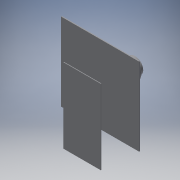
# Autodesk Inventor part: base1
Saved by Autodesk Inventor 2019 (Build 230136000, 136)
## iProperties
Created: 2019-05-27
Part Number: base1
Material: Generic
Document SubType Name: Modeling
Designer: felix
Density: 1 g/cm^3
Appearance: Default
Mass: 50923.6 g
Surface Area: 49527 cm^2
Volume: 50923.6 cm^3
Author: felix
Autodesk Inventor part; units mm, degrees
sketch "Sketch1" plane through (0, 0, 0) normal (0, 0, 1) x (1, 0, 0)
  circle A0 centre (0, 0) radius 130.5
  dimension "d0" = 261
  constraints: 1 centre point, 1 coincident
  measures "d0" diameter of A0
extrude "Extrusion1" add sketch "Sketch1" along normal blind 30 and the other way blind 95
sketch "Sketch2" plane through (0, 0, 30) normal (0, 0, 1) x (1, 0, 0)
  circle A0 centre (0, 0) radius 172.5
  dimension "d3" = 345
  constraints: 1 centre point, 1 coincident
  measures "d3" diameter of A0
extrude "Extrusion2" add sketch "Sketch2" along normal blind 125 and the other way blind 52.75
sketch "Sketch3" plane through (0, 0, 155) normal (0, 0, 1) x (1, 0, 0)
  line L0 (-920, 350) -> (330, 350)
  line L1 (330, 350) -> (330, -900)
  line L2 (330, -900) -> (-920, -900)
  line L3 (-920, -900) -> (-920, 350)
  point P0 (0, 0)
  dimension "d8" = 920
  dimension "d9" = 1250
  dimension "d10" = 900
  dimension "d11" = 1250
  constraints: 8 end point, 2 parallel, 1 horizontal, 1 perpendicular
  measures "d8" distance from line of point (0, 0) L3
  measures "d9" distance of L0.end L1.end
  measures "d10" vertical distance of point (0, 0) L2.end
  measures "d11" distance of L1.end L2.end
extrude "Extrusion3" add sketch "Sketch3" along normal blind 15
sketch "Sketch5" plane through (0, 0, 155) normal (0, 0, -1) x (-1, 0, 0)
  line L0 (-315, -885) -> (905, -885)
  line L1 (905, -885) -> (905, 335)
  line L2 (905, 335) -> (-315, 335)
  line L3 (-315, 335) -> (-315, -885)
  line L4 (590, -885) -> (590, -515)
  line L5 (590, -515) -> (905, -515)
  line L6 (590, -515) -> (590, -105)
  line L7 (590, -105) -> (905, -105)
  line L8 (590, -105) -> (590, 335)
  line L9 (-315, -335) -> (590, -335)
  point P0 (0, 0)
  dimension "d14" = 885
  dimension "d15" = 335
  dimension "d16" = 315
  dimension "d17" = 905
  dimension "d18" = 370
  dimension "d19" = 315
  dimension "d20" = 440
  dimension "d22" = 335
  constraints: 20 end point, 7 point on line, 5 perpendicular, 2 parallel, 1 horizontal, 1 vertical
  measures "d14" vertical distance of L0.start point (0, 0)
  measures "d15" vertical distance of point (0, 0) L2.end
  measures "d16" distance from line of L3 point (0, 0)
  measures "d17" distance from line of L1 point (0, 0)
  measures "d18" distance of L4.start L4.end
  measures "d19" distance of L4.end L5.end
  measures "d20" distance of L6.end L8.end
  measures "d22" distance from line of point (0, 0) L9
ref_plane "Work Plane1" through (-895, -900, 155) normal (-1, 0, 0) x (0, 0, 1)
sketch "Sketch7" plane through (-895, -900, 155) normal (-1, 0, 0) x (0, 0, 1)
  line L0 (0, 0) -> (15, 0) projected
  line L1 (0, 0) -> (0, 1250) projected
  line L2 (35, 25) -> (1005, 25)
  line L3 (1005, 25) -> (1005, 1225)
  line L4 (1005, 1225) -> (35, 1225)
  line L5 (35, 1225) -> (35, 25)
  line L6 (35, 625) -> (600, 625)
  line L7 (600, 25) -> (600, 1225)
  point P0 (-155, 900)
  dimension "d24" = 25
  dimension "d25" = 35
  dimension "d26" = 1200
  dimension "d27" = 970
  dimension "d78" = 600
  constraints: 12 end point, 2 horizontal, 2 midpoint, 2 parallel, 2 point on line, 1 perpendicular, 1 vertical
  measures "d24" distance between parallel lines of L2 L0
  measures "d25" distance between parallel lines of L1 L5
  measures "d26" distance of L2.end L3.end
  measures "d27" distance of L3.end L4.end
  measures "d78" distance between parallel lines of L7 L1
ref_plane "Work Plane2" through (-920, -875, 155) normal (0, -1, 0) x (1, 0, 0)
sketch "Sketch8" plane through (-920, -875, 155) normal (0, -1, 0) x (1, 0, 0)
  line L0 (1250, 0) -> (1250, 15) projected
  line L1 (1250, 0) -> (0, 0) projected
  line L2 (1225, 35) -> (25, 35)
  line L3 (25, 35) -> (25, 1005)
  line L4 (25, 1005) -> (1225, 1005)
  line L5 (1225, 1005) -> (1225, 35)
  line L6 (1225, 600) -> (25, 600)
  line L7 (625, 600) -> (625, 35)
  line L8 (25, 285) -> (625, 35)
  line L9 (1225, 285) -> (625, 35)
  point P0 (920, -155)
  dimension "d29" = 25
  dimension "d30" = 35
  dimension "d31" = 1200
  dimension "d32" = 970
  dimension "d33" = 600
  dimension "d66" = 0
  dimension "d67" = 250
  dimension "d68" = 250
  constraints: 16 end point, 5 point on line, 2 horizontal, 2 midpoint, 2 parallel, 1 perpendicular
  measures "d29" distance between parallel lines of L5 L0
  measures "d30" distance between parallel lines of L1 L2
  measures "d31" distance of L3.end L4.end
  measures "d32" distance of L2.end L3.end
  measures "d33" distance between parallel lines of L6 L1
  measures "d66" distance of L8.end L7.end
  measures "d67" distance of L8.start L2.end
  measures "d68" distance of L9.start L2.start
ref_plane "Work Plane3" through (-920, 325, 155) normal (0, 1, 0) x (1, 0, 0)
sketch "Sketch9" plane through (-920, 325, 155) normal (0, 1, 0) x (1, 0, 0)
  line L0 (25, -35) -> (1225, -35)
  line L1 (1225, -35) -> (1225, -1005)
  line L2 (1225, -1005) -> (25, -1005)
  line L3 (25, -1005) -> (25, -35)
  line L4 (0, 0) -> (0, -15) projected
  line L5 (0, 0) -> (1250, 0) projected
  line L6 (25, -600) -> (1225, -600)
  line L7 (625, -600) -> (625, -35)
  line L8 (25, -285) -> (625, -35)
  line L9 (625, -35) -> (1225, -285)
  point P0 (920, 155)
  dimension "d35" = 25
  dimension "d36" = 35
  dimension "d37" = 1200
  dimension "d38" = 970
  dimension "d39" = 600
  dimension "d69" = 250
  dimension "d70" = 250
  constraints: 16 end point, 4 point on line, 2 midpoint, 2 parallel, 2 perpendicular, 1 horizontal
  measures "d35" distance between parallel lines of L3 L4
  measures "d36" distance between parallel lines of L5 L0
  measures "d37" distance of L1.end L2.end
  measures "d38" distance of L0.end L1.end
  measures "d39" distance between parallel lines of L6 L5
  measures "d69" distance of L8.start L0.start
  measures "d70" distance of L9.end L0.end
ref_plane "Work Plane4" through (305, -900, 155) normal (1, 0, 0) x (0, 0, -1)
sketch "Sketch10" plane through (305, -900, 155) normal (1, 0, 0) x (0, 0, -1)
  line L0 (-35, 1225) -> (-1005, 1225)
  line L1 (-1005, 1225) -> (-1005, 25)
  line L2 (-1005, 25) -> (-35, 25)
  line L3 (-35, 25) -> (-35, 1225)
  line L4 (0, 1250) -> (-15, 1250) projected
  line L5 (0, 1250) -> (0, 0) projected
  line L6 (-600, 1225) -> (-600, 25)
  line L7 (-600, 625) -> (-35, 625)
  line L8 (-285, 25) -> (-35, 625)
  line L9 (-35, 625) -> (-285, 1225)
  point P0 (155, 900)
  dimension "d41" = 25
  dimension "d42" = 35
  dimension "d43" = 1200
  dimension "d44" = 970
  dimension "d45" = 600
  dimension "d71" = 250
  dimension "d72" = 250
  constraints: 16 end point, 4 point on line, 2 midpoint, 2 parallel, 1 horizontal, 1 perpendicular, 1 vertical
  measures "d41" distance between parallel lines of L0 L4
  measures "d42" distance between parallel lines of L5 L3
  measures "d43" distance of L0.end L1.end
  measures "d44" distance of L1.end L2.end
  measures "d45" distance between parallel lines of L6 L5
  measures "d71" distance of L9.end L0.start
  measures "d72" distance of L8.start L2.end
ref_plane "Work Plane5" through (0, 0, 755) normal (0, 0, 1) x (1, 0, 0)
sketch "Sketch11" plane through (0, 0, 755) normal (0, 0, 1) x (1, 0, 0)
  line L0 (305, 325) -> (-295, 325)
  line L1 (-295, 325) -> (-295, -875)
  line L2 (-295, -875) -> (305, -875)
  line L3 (305, -875) -> (305, 325)
  line L4 (330, 350) -> (-920, 350) projected
  line L5 (330, -900) -> (330, 350) projected
  line L6 (-895, -275) -> (305, -275)
  line L7 (-295, -875) -> (-895, -875)
  line L8 (-920, 350) -> (-920, -900) projected
  line L9 (-295, 325) -> (-895, 325)
  line L10 (-895, 325) -> (-895, -875)
  point P0 (0, 0)
  point P1 (-295, -275)
  point P2 (-920, -900)
  dimension "d47" = 25
  dimension "d48" = 25
  dimension "d49" = 1200
  dimension "d50" = 625
  dimension "d79" = 600
  dimension "d80" = 600
  constraints: 16 end point, 4 midpoint, 3 parallel, 1 horizontal, 1 perpendicular, 1 point on line, 1 other
  measures "d47" distance between parallel lines of L0 L4
  measures "d48" distance between parallel lines of L5 L3
  measures "d49" distance of L0.end L1.end
  measures "d50" distance between parallel lines of L1 L5
  measures "d79" distance of L1.end L7.end
  measures "d80" distance of L0.end L9.end
sketch "Sketch13" plane through (0, 0, -95) normal (0, 0, -1) x (-1, 0, 0)
  point P0 (0, 0)
  point P1 (-0.2124, -84.047)
hole "Hole1" at (0.2124, -84.047, -95) direction (0, 0, 1) diameter 30 depth 190 tip angle 160
ref_plane "Work Plane8" through (0, -172.5, 30) normal (0, -1, 0) x (1, 0, 0)
sketch "Sketch14" plane through (0, -172.5, 30) normal (0, -1, 0) x (1, 0, 0)
  circle A0 centre (0, 60) radius 15
  point P0 (0, -30)
  dimension "d60" = 30
  dimension "d61" = 90
  constraints: 1 centre point, 1 vertical alignment
  measures "d60" diameter of A0
  measures "d61" distance of A0.centre point (0, -30)
extrude "Extrusion4" cut sketch "Sketch14" against normal blind 105
extrude "Extrusion5" add sketch "Sketch11" along normal mid plane 10 contours L3 L2 L1 L6
extrude "Extrusion6" add sketch "Sketch11" along normal mid plane 10 contours L3 L6 L1 L0
extrude "Extrusion7" add sketch "Sketch11" along normal mid plane 10 contours L1 L6 L10 L9 | L1 L7 L10 L6
body "Solid1"
